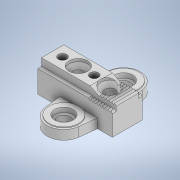
# Autodesk Inventor part: nkosi_zawias
Saved by Autodesk Inventor 2020.3 (Build 243373000, 373)
## iProperties
Created: 2020-08-23
Part Number: nkosi_zawias
Material: Generic
Document SubType Name: Modeling
Designer: nawyk
Density: 1 g/cm^3
Appearance: Default
Author: nawyk
Autodesk Inventor part; units mm, degrees
ref_plane "YZ Plane" through (0, 0, 0) normal (1, 0, 0) x (0, 1, 0)
ref_plane "XZ Plane" through (0, 0, 0) normal (0, 1, 0) x (-1, 0, 0)
ref_plane "XY Plane" through (0, 0, 0) normal (0, 0, 1) x (1, 0, 0)
sketch "Sketch1" plane through (0, 0, 0) normal (0, 1, 0) x (-1, 0, 0)
  line L0 (0, 0) -> (40, 0)
  line L1 (40, 0) -> (40, -16)
  line L2 (40, -16) -> (0, -16)
  line L3 (0, -16) -> (0, 0)
  line L4 (0, 0) -> (19, 0)
  line L5 (0, -8) -> (18, -8)
  line L6 (18, -8) -> (18, -24)
  line L7 (18, -8) -> (18, 8)
  circle A0 centre (18, -24) radius 3.5
  circle A1 centre (18, 8) radius 3.3496
  line L8 (18, -16) -> (28, -16)
  line L9 (28, -16) -> (28, -33)
  line L10 (28, -33) -> (18, -33)
  line L11 (18, -33) -> (18, -16)
  line L12 (18, -33) -> (8, -33)
  line L13 (8, -33) -> (8, -16)
  line L14 (8, -16) -> (18, -16)
  line L15 (18, -16) -> (18, -33)
  line L16 (18, 0) -> (28, 0)
  line L17 (18, 0) -> (8, 0)
  line L18 (8, 0) -> (8, 17)
  line L19 (8, 17) -> (18, 17)
  line L20 (18, 17) -> (18, 0)
  line L21 (18, 0) -> (28, 0)
  line L22 (28, 0) -> (28, 17)
  line L23 (28, 17) -> (18, 17)
  line L24 (18, 17) -> (18, 0)
  dimension "d0" = 40
  dimension "d1" = 16
  dimension "d3" = 18
  dimension "d4" = 16
  dimension "d5" = 16
  dimension "d6" = 7
  dimension "d9" = 10
  dimension "d10" = 17
  dimension "d11" = 10
  dimension "d13" = 10
  dimension "d14" = 17
  dimension "d15" = 10
  constraints: 50 end point, 10 parallel, 7 horizontal, 5 perpendicular, 3 midpoint, 2 centre point, 2 coincident, 2 point on line, 2 vertical
  measures "d0" distance of L1.end L2.end
  measures "d1" distance of L0.end L1.end
  measures "d3" distance of L5.start L5.end
  measures "d4" distance of L5.end L6.end
  measures "d5" distance of L5.end L7.end
  measures "d6" diameter of A0
  measures "d9" distance of L9.end L10.end
  measures "d10" distance of L8.end L9.end
  measures "d11" distance of L13.end L14.end
  measures "d13" distance of L18.end L19.end
  measures "d14" distance of L17.end L18.end
  measures "d15" distance of L23.end L22.end
extrude "Extrusion1" add sketch "Sketch1" along normal blind 5 contours L0 L7 L5 L3 | L18 L19 L20 A1 L7 L0 | L5 L6 L2 L3 | L7 A1 L20 L23 L22 L0 | L0 L1 L2 L6 L7 | L2 L6 A0 L11 L12 L13 | L2 L9 L10 L11 A0 L6
sketch "Sketch2" plane through (0, 5, 0) normal (0, 1, 0) x (1, 0, 0)
  circle A0 centre (-18, 24) radius 3.5 projected
  circle A1 centre (-18, 24) radius 9
  circle A2 centre (-18, -8) radius 3.3496 projected
  circle A3 centre (-18, -8) radius 9
  line L0 (-28, -17) -> (-8, -17) projected
  line L1 (-28, 33) -> (-28, 16) projected
  line L2 (-28, 16) -> (-26.9387, 25.0484)
  line L3 (0, 16) -> (-8, 16) projected
  line L4 (-8, 16) -> (-9.0613, 25.0484)
  line L5 (-8, -17) -> (-8, 0) projected
  line L6 (-8, 0) -> (-9.0613, -9.0484)
  line L7 (-28, 0) -> (-26.9387, -9.0484)
  line L8 (-40, 0) -> (-28, 0) projected
  line L9 (-28, 0) -> (-28, -17)
  line L10 (-28, -17) -> (-8, -17)
  line L11 (-8, -17) -> (-8, 0)
  line L12 (-28, 16) -> (-28, 33)
  line L13 (-8, 33) -> (-28, 33) projected
  line L14 (-28, 33) -> (-8, 33)
  line L15 (-8, 16) -> (-8, 33) projected
  line L16 (-8, 33) -> (-8, 16)
  point P0 (0, 0)
  point P1 (-18, 33)
  point P2 (-18, -17)
  constraints: 20 end point, 4 equal length, 4 point on circle, 3 tangent, 2 centre point, 2 coincident, 2 perpendicular, 1 point on line, 1 vertical
extrude "Extrusion2" cut sketch "Sketch2" against normal up to surface (5 mm away) contours A1 L13 L15 L4 | L2 L1 L13 A1 | A3 L0 L9 L7 | L6 L5 L0 A3
sketch "Sketch3" plane through (0, 5, 0) normal (0, 1, 0) x (1, 0, 0)
  circle A0 centre (-18, -8) radius 3.3496 projected
  circle A1 centre (-18, -8) radius 5
  circle A2 centre (-18, 24) radius 3.5 projected
  circle A3 centre (-18, 24) radius 5
  point P0 (0, 0)
  dimension "d20" = 10
  dimension "d21" = 10
  constraints: 2 centre point, 2 coincident
  measures "d20" diameter of A1
  measures "d21" diameter of A3
extrude "Extrusion3" cut sketch "Sketch3" against normal blind 2
sketch "Sketch4" plane through (0, 5, 0) normal (0, 1, 0) x (1, 0, 0)
  circle A0 centre (-18, 24) radius 5 projected
  circle A1 centre (-18, 24) radius 5
  circle A2 centre (-18, -8) radius 5 projected
  circle A3 centre (-18, -8) radius 5
  line L0 (-40, 0) -> (-28, 0) projected
  line L1 (0, 16) -> (-8, 16) projected
  line L2 (-40, 0) -> (0, 0)
  line L3 (0, 0) -> (0, 16)
  line L4 (0, 16) -> (-40, 16)
  line L5 (-40, 16) -> (-40, 0)
  circle A4 centre (-18, -8) radius 8
  circle A5 centre (-18, 24) radius 8
  constraints: 8 end point, 4 centre point, 4 coincident, 2 parallel, 2 tangent, 1 horizontal, 1 perpendicular
extrude "Extrusion4" add sketch "Sketch4" along normal blind 0.5 contours A5 | A4
sketch "Sketch5" plane through (0, 0, 0) normal (0, -1, 0) x (1, 0, 0)
  line L0 (-28, -16) -> (-40, -16) projected
  line L1 (0, 0) -> (0, -16) projected
  line L2 (-40, -16) -> (0, -16)
  line L3 (0, -16) -> (0, 0)
  line L4 (0, 0) -> (-40, 0)
  line L5 (-40, 0) -> (-40, -16)
  constraints: 8 end point, 2 parallel, 1 horizontal, 1 perpendicular
extrude "Extrusion5" add sketch "Sketch5" against normal blind 12
sketch "Sketch6" plane through (0, 12, 0) normal (0, 1, 0) x (1, 0, 0)
  line L0 (0, 0) -> (0, 16) projected
  line L1 (-40, 0) -> (0, 0)
  line L2 (0, 0) -> (0, 2)
  line L3 (0, 2) -> (-40, 2)
  line L4 (-40, 2) -> (-40, 0)
  line L5 (-40, 16) -> (0, 16)
  line L6 (0, 16) -> (0, 14)
  line L7 (0, 14) -> (-40, 14)
  line L8 (-40, 14) -> (-40, 16)
  line L9 (-40, 2) -> (0, 2)
  line L10 (0, 2) -> (0, 14)
  line L11 (0, 14) -> (-40, 14)
  line L12 (-40, 14) -> (-40, 2)
  dimension "d28" = 2
  dimension "d29" = 2
  constraints: 24 end point, 6 parallel, 3 horizontal, 3 perpendicular, 2 point on line
  measures "d28" distance of L2.end L1.end
  measures "d29" distance of L5.end L6.end
extrude "Extrusion6" add sketch "Sketch6" along normal blind 4 contours L3 L12 L7 L0
sketch "Sketch7" plane through (0, 12, -14) normal (0, 0, -1) x (-1, 0, 0)
  line L0 (0, -12) -> (0, 0) projected
  line L1 (40, 0) -> (40, 4) projected
  line L2 (0, 0) -> (40, 0)
  line L3 (40, 0) -> (40, 2.5)
  line L4 (40, 2.5) -> (0, 2.5)
  line L5 (0, 2.5) -> (0, 0)
  line L6 (40, 4) -> (14, 4)
  line L7 (14, 4) -> (14, 2.5)
  line L8 (14, 2.5) -> (40, 2.5)
  line L9 (40, 2.5) -> (40, 4)
  line L10 (40, 4) -> (0, 4) projected
  line L11 (0, 2.5) -> (9, 2.5)
  line L12 (9, 2.5) -> (9, 4)
  line L13 (9, 4) -> (0, 4)
  line L14 (0, 4) -> (0, 2.5)
  line L15 (9, 2.5) -> (14, 4)
  line L16 (14, 4) -> (0, 4)
  dimension "d32" = 2.5
  dimension "d33" = 26
  dimension "d34" = 9
  constraints: 28 end point, 6 parallel, 3 horizontal, 3 perpendicular, 3 point on line, 1 collinear
  measures "d32" distance of L3.end L2.end
  measures "d33" distance of L8.end L7.end
  measures "d34" distance of L13.end L12.end
extrude "Extrusion7" cut sketch "Sketch7" against normal up to surface (12 mm away) contours L14 L10 L12 L4 | L15 L12 L10
sketch "Sketch8" plane through (0, 12, -14) normal (0, 0, -1) x (-1, 0, 0)
  line L0 (0, 0) -> (0, 2.5) projected
  line L1 (0, 2.5) -> (9, 2.5)
  line L2 (9, 2.5) -> (9, 1.5)
  line L3 (9, 1.5) -> (0, 1.5)
  line L4 (0, 1.5) -> (0, 2.5)
  line L5 (0, 2.5) -> (0.75, 2.5)
  line L6 (0.75, 2.5) -> (0.75, 1.5)
  line L7 (0.75, 1.5) -> (0, 1.5)
  line L8 (0, 1.5) -> (0, 2.5)
  line L9 (9, 2.5) -> (0, 2.5) projected
  line L10 (0.75, 1.5) -> (1.5, 1.5)
  line L11 (1.5, 1.5) -> (1.5, 2.5)
  line L12 (1.5, 2.5) -> (0.75, 2.5)
  line L13 (0.75, 2.5) -> (0.75, 1.5)
  line L14 (1.5, 1.5) -> (2.25, 1.5)
  line L15 (2.25, 1.5) -> (2.25, 2.5)
  line L16 (2.25, 2.5) -> (1.5, 2.5)
  line L17 (1.5, 2.5) -> (1.5, 1.5)
  line L18 (2.25, 1.5) -> (3, 1.5)
  line L19 (3, 1.5) -> (3, 2.5)
  line L20 (3, 2.5) -> (2.25, 2.5)
  line L21 (2.25, 2.5) -> (2.25, 1.5)
  line L22 (3, 1.5) -> (3.75, 1.5)
  line L23 (3.75, 1.5) -> (3.75, 2.5)
  line L24 (3.75, 2.5) -> (3, 2.5)
  line L25 (3, 2.5) -> (3, 1.5)
  line L26 (3.75, 1.5) -> (4.5, 1.5)
  line L27 (4.5, 1.5) -> (4.5, 2.5)
  line L28 (4.5, 2.5) -> (3.75, 2.5)
  line L29 (3.75, 2.5) -> (3.75, 1.5)
  line L30 (4.5, 1.5) -> (5.25, 1.5)
  line L31 (5.25, 1.5) -> (5.25, 2.5)
  line L32 (5.25, 2.5) -> (4.5, 2.5)
  line L33 (4.5, 2.5) -> (4.5, 1.5)
  line L34 (5.25, 1.5) -> (6, 1.5)
  line L35 (6, 1.5) -> (6, 2.5)
  line L36 (6, 2.5) -> (5.25, 2.5)
  line L37 (5.25, 2.5) -> (5.25, 1.5)
  line L38 (6, 1.5) -> (6.75, 1.5)
  line L39 (6.75, 1.5) -> (6.75, 2.5)
  line L40 (6.75, 2.5) -> (6, 2.5)
  line L41 (6, 2.5) -> (6, 1.5)
  line L42 (6.75, 1.5) -> (7.5, 1.5)
  line L43 (7.5, 1.5) -> (7.5, 2.5)
  line L44 (7.5, 2.5) -> (6.75, 2.5)
  line L45 (6.75, 2.5) -> (6.75, 1.5)
  line L46 (7.5, 1.5) -> (8.25, 1.5)
  line L47 (8.25, 1.5) -> (8.25, 2.5)
  line L48 (8.25, 2.5) -> (7.5, 2.5)
  line L49 (7.5, 2.5) -> (7.5, 1.5)
  line L50 (9, 2.5) -> (14, 4) projected
  line L51 (8.25, 1.5) -> (9, 1.5)
  line L52 (9, 1.5) -> (9, 2.5)
  line L53 (9, 2.5) -> (8.25, 2.5)
  line L54 (8.25, 2.5) -> (8.25, 1.5)
  line L55 (0, 1.5) -> (0.75, 2.5)
  line L56 (9, 1.5) -> (8.25, 2.5)
  line L57 (7.5, 1.5) -> (6.75, 2.5)
  line L58 (6, 1.5) -> (5.25, 2.5)
  line L59 (4.5, 1.5) -> (3.75, 2.5)
  line L60 (3, 1.5) -> (2.25, 2.5)
  line L61 (1.5, 1.5) -> (0.75, 2.5)
  line L62 (1.5, 1.5) -> (2.25, 2.5)
  line L63 (3, 1.5) -> (3.75, 2.5)
  line L64 (4.5, 1.5) -> (5.25, 2.5)
  line L65 (6, 1.5) -> (6.75, 2.5)
  line L66 (7.5, 1.5) -> (8.25, 2.5)
  line L67 (14, 4) -> (40, 4) projected
  line L68 (14, 4) -> (9, 1.5)
  line L69 (14, 4) -> (9, 2.5)
  line L70 (9, 2.5) -> (0, 2.5)
  line L71 (0, 1.5) -> (0, 2.5)
  point P0 (0, -12)
  point P1 (0, 1.5)
  constraints: 136 end point, 34 equal length, 14 horizontal, 14 perpendicular, 11 point on line, 1 midpoint
extrude "Extrusion8" cut sketch "Sketch8" against normal up to surface (12 mm away) contours L0 L1 L55 | L1 L11 L61 | L11 L1 L62 | L1 L19 L60 | L19 L1 L63 | L1 L27 L59 | L27 L1 L64 | L1 L35 L58 | L35 L1 L65 | L1 L43 L57 | L43 L1 L66 | L1 L2 L56 | L2 L50 L68
sketch "Sketch9" plane through (-28, 0, -16) normal (0, 0, -1) x (-1, 0, 0)
  line L0 (-28, 12) -> (-28, 13.5) projected
  line L1 (-28, 12) -> (-16, 12)
  line L2 (-16, 12) -> (-16, 11)
  line L3 (-16, 11) -> (-28, 11)
  line L4 (-28, 11) -> (-28, 12)
  line L5 (-28, 12) -> (12, 12) projected
  line L6 (-16, 11) -> (-16.75, 11)
  line L7 (-16.75, 11) -> (-16.75, 12)
  line L8 (-16.75, 12) -> (-16, 12)
  line L9 (-16, 12) -> (-16, 11)
  line L10 (-16.75, 11) -> (-17.5, 11)
  line L11 (-17.5, 11) -> (-17.5, 12)
  line L12 (-17.5, 12) -> (-16.75, 12)
  line L13 (-16.75, 12) -> (-16.75, 11)
  line L14 (-17.5, 11) -> (-18.25, 11)
  line L15 (-18.25, 11) -> (-18.25, 12)
  line L16 (-18.25, 12) -> (-17.5, 12)
  line L17 (-17.5, 12) -> (-17.5, 11)
  line L18 (-18.25, 11) -> (-19, 11)
  line L19 (-19, 11) -> (-19, 12)
  line L20 (-19, 12) -> (-18.25, 12)
  line L21 (-18.25, 12) -> (-18.25, 11)
  line L22 (-19, 11) -> (-19.75, 11)
  line L23 (-19.75, 11) -> (-19.75, 12)
  line L24 (-19.75, 12) -> (-19, 12)
  line L25 (-19, 12) -> (-19, 11)
  line L26 (-19.75, 11) -> (-20.5, 11)
  line L27 (-20.5, 11) -> (-20.5, 12)
  line L28 (-20.5, 12) -> (-19.75, 12)
  line L29 (-19.75, 12) -> (-19.75, 11)
  line L30 (-20.5, 11) -> (-21.25, 11)
  line L31 (-21.25, 11) -> (-21.25, 12)
  line L32 (-21.25, 12) -> (-20.5, 12)
  line L33 (-20.5, 12) -> (-20.5, 11)
  line L34 (-21.25, 11) -> (-22, 11)
  line L35 (-22, 11) -> (-22, 12)
  line L36 (-22, 12) -> (-21.25, 12)
  line L37 (-21.25, 12) -> (-21.25, 11)
  line L38 (-22, 11) -> (-22.75, 11)
  line L39 (-22.75, 11) -> (-22.75, 12)
  line L40 (-22.75, 12) -> (-22, 12)
  line L41 (-22, 12) -> (-22, 11)
  line L42 (-22.75, 11) -> (-23.5, 11)
  line L43 (-23.5, 11) -> (-23.5, 12)
  line L44 (-23.5, 12) -> (-22.75, 12)
  line L45 (-22.75, 12) -> (-22.75, 11)
  line L46 (-23.5, 11) -> (-24.25, 11)
  line L47 (-24.25, 11) -> (-24.25, 12)
  line L48 (-24.25, 12) -> (-23.5, 12)
  line L49 (-23.5, 12) -> (-23.5, 11)
  line L50 (-24.25, 11) -> (-25, 11)
  line L51 (-25, 11) -> (-25, 12)
  line L52 (-25, 12) -> (-24.25, 12)
  line L53 (-24.25, 12) -> (-24.25, 11)
  line L54 (-25, 11) -> (-25.75, 11)
  line L55 (-25.75, 11) -> (-25.75, 12)
  line L56 (-25.75, 12) -> (-25, 12)
  line L57 (-25, 12) -> (-25, 11)
  line L58 (-25.75, 11) -> (-26.5, 11)
  line L59 (-26.5, 11) -> (-26.5, 12)
  line L60 (-26.5, 12) -> (-25.75, 12)
  line L61 (-25.75, 12) -> (-25.75, 11)
  line L62 (-26.5, 11) -> (-27.25, 11)
  line L63 (-27.25, 11) -> (-27.25, 12)
  line L64 (-27.25, 12) -> (-26.5, 12)
  line L65 (-26.5, 12) -> (-26.5, 11)
  line L66 (-28, 0) -> (-28, 12) projected
  line L67 (-27.25, 11) -> (-28, 11)
  line L68 (-28, 11) -> (-28, 12)
  line L69 (-28, 12) -> (-27.25, 12)
  line L70 (-27.25, 12) -> (-27.25, 11)
  line L71 (-16, 11) -> (-16.75, 12)
  line L72 (-16.75, 12) -> (-17.5, 11)
  line L73 (-17.5, 11) -> (-18.25, 12)
  line L74 (-18.25, 12) -> (-19, 11)
  line L75 (-19, 11) -> (-19.75, 12)
  line L76 (-19.75, 12) -> (-20.5, 11)
  line L77 (-20.5, 11) -> (-21.25, 12)
  line L78 (-21.25, 12) -> (-22, 11)
  line L79 (-22, 11) -> (-22.75, 12)
  line L80 (-22.75, 12) -> (-23.5, 11)
  line L81 (-23.5, 11) -> (-24.25, 12)
  line L82 (-24.25, 12) -> (-25, 11)
  line L83 (-25, 11) -> (-25.75, 12)
  line L84 (-25.75, 12) -> (-26.5, 11)
  line L85 (-26.5, 11) -> (-27.25, 12)
  line L86 (-27.25, 12) -> (-28, 11)
  line L87 (-16, 11) -> (-15.25, 11)
  line L88 (-15.25, 11) -> (-15.25, 12)
  line L89 (-15.25, 12) -> (-16, 12)
  line L90 (-16, 12) -> (-16, 11)
  line L91 (-16, 11) -> (-15.25, 12)
  dimension "d55" = 0.75
  dimension "d56" = 0.75
  dimension "d57" = 0.75
  dimension "d58" = 0.75
  dimension "d59" = 0.75
  dimension "d60" = 0.75
  dimension "d61" = 0.75
  dimension "d62" = 0.75
  dimension "d63" = 0.75
  dimension "d64" = 0.75
  dimension "d65" = 0.75
  dimension "d66" = 0.75
  dimension "d67" = 0.75
  dimension "d68" = 0.75
  dimension "d69" = 0.75
  dimension "d70" = 0.75
  constraints: 176 end point, 36 parallel, 18 horizontal, 17 perpendicular, 1 point on line, 1 vertical, 20 other
  measures "d55" distance of L7.end L8.end
  measures "d56" distance of L11.end L12.end
  measures "d57" distance of L15.end L16.end
  measures "d58" distance of L19.end L20.end
  measures "d59" distance of L23.end L24.end
  measures "d60" distance of L27.end L28.end
  measures "d61" distance of L31.end L32.end
  measures "d62" distance of L35.end L36.end
  measures "d63" distance of L39.end L40.end
  measures "d64" distance of L43.end L44.end
  measures "d65" distance of L47.end L48.end
  measures "d66" distance of L51.end L52.end
  measures "d67" distance of L55.end L56.end
  measures "d68" distance of L59.end L60.end
  measures "d69" distance of L63.end L64.end
  measures "d70" distance of L89.end L88.end
extrude "Extrusion9" cut sketch "Sketch9" against normal up to surface (2 mm away) contours L1 L86 L4 | L1 L59 L85 | L1 L84 L59 | L1 L51 L83 | L1 L82 L51 | L1 L43 L81 | L1 L80 L43 | L1 L35 L79 | L1 L78 L35 | L1 L27 L77 | L1 L76 L27 | L1 L19 L75 | L1 L74 L19 | L1 L11 L73 | L1 L72 L11 | L1 L2 L71 | L5 L91 L2
sketch "Sketch10" plane through (-40, 0, 0) normal (0, 0, 1) x (1, 0, 0)
  line L0 (40, 12) -> (40, 13.5) projected
  line L1 (40, 12) -> (28, 12)
  line L2 (28, 12) -> (28, 11)
  line L3 (28, 11) -> (40, 11)
  line L4 (40, 11) -> (40, 12)
  line L5 (28, 11) -> (28.75, 12) projected
  line L6 (28.75, 12) -> (29.5, 11) projected
  line L7 (28, 11) -> (28.75, 12)
  line L8 (28.75, 12) -> (29.5, 11)
  line L9 (29.5, 11) -> (30.25, 12) projected
  line L10 (29.5, 11) -> (30.25, 12)
  line L11 (31, 11) -> (31.75, 12) projected
  line L12 (30.25, 12) -> (31, 11)
  line L13 (31, 11) -> (31.75, 12)
  line L14 (31.75, 12) -> (32.5, 11) projected
  line L15 (31.75, 12) -> (32.5, 11)
  line L16 (32.5, 11) -> (33.25, 12) projected
  line L17 (32.5, 11) -> (33.25, 12)
  line L18 (33.25, 12) -> (34, 11) projected
  line L19 (33.25, 12) -> (34, 11)
  line L20 (34.75, 12) -> (35.5, 11) projected
  line L21 (34, 11) -> (34.75, 12)
  line L22 (35.5, 11) -> (36.25, 12) projected
  line L23 (34.75, 12) -> (35.5, 11)
  line L24 (35.5, 11) -> (36.25, 12)
  line L25 (36.25, 12) -> (37, 11) projected
  line L26 (36.25, 12) -> (37, 11)
  line L27 (37, 11) -> (37.75, 12) projected
  line L28 (37, 11) -> (37.75, 12)
  line L29 (38.5, 11) -> (39.25, 12) projected
  line L30 (37.75, 12) -> (38.5, 11)
  line L31 (38.5, 11) -> (39.25, 12)
  line L32 (39.25, 12) -> (40, 11) projected
  line L33 (39.25, 12) -> (40, 11)
  line L34 (40, 11) -> (40, 12)
  line L35 (40, 12) -> (0, 12) projected
  line L36 (40, 12) -> (28, 12)
  line L37 (27.25, 12) -> (28, 11) projected
  line L38 (28, 11) -> (27.25, 12)
  line L39 (27.25, 12) -> (28, 12)
  point P0 (40, 0)
  constraints: 44 end point, 9 collinear, 9 parallel, 2 vertical, 1 horizontal, 7 other
extrude "Extrusion10" cut sketch "Sketch10" against normal up to surface (2 mm away) contours L4 L32 L1 | L29 L30 L1 | L27 L25 L1 | L22 L20 L1 | L21 L18 L1 | L16 L14 L1 | L11 L12 L1 | L9 L6 L1 | L5 L2 L1 | L2 L37 L35
sketch "Sketch11" plane through (0, 16, 0) normal (0, 1, 0) x (1, 0, 0)
  line L0 (-40, 14) -> (-40, 2) projected
  line L1 (-40, 8) -> (-34.75, 8)
  circle A0 centre (-34.75, 8) radius 2.25
  line L2 (-34.75, 8) -> (-17.75, 8)
  circle A1 centre (-17.75, 8) radius 2.25
  circle A2 centre (-26.25, 8) radius 2.825
  line L3 (-26.25, 8) -> (-9.25, 8)
  circle A3 centre (-9.25, 8) radius 2.825
  point P0 (0, 0)
  dimension "d77" = 5.25
  dimension "d78" = 4.5
  dimension "d79" = 17
  dimension "d80" = 4.5
  dimension "d81" = 5.65
  dimension "d82" = 17
  dimension "d83" = 5.65
  constraints: 6 end point, 4 centre point, 3 coincident, 2 horizontal, 2 midpoint, 1 point on line
  measures "d77" distance of L1.start L1.end
  measures "d78" diameter of A0
  measures "d79" distance of L2.start L2.end
  measures "d80" diameter of A1
  measures "d81" diameter of A2
  measures "d82" distance of L3.start L3.end
  measures "d83" diameter of A3
extrude "Extrusion11" cut sketch "Sketch11" against normal up to surface (16 mm away)
sketch "Sketch12" plane through (0, 16, 0) normal (0, 1, 0) x (1, 0, 0)
  circle A0 centre (-26.25, 8) radius 2.825 projected
  circle A1 centre (-26.25, 8) radius 5
  circle A2 centre (-9.25, 8) radius 2.825 projected
  circle A3 centre (-9.25, 8) radius 5
  point P0 (0, 0)
  dimension "d86" = 10
  dimension "d87" = 10
  constraints: 2 centre point, 2 coincident
  measures "d86" diameter of A1
  measures "d87" diameter of A3
extrude "Extrusion12" cut sketch "Sketch12" against normal blind 1.5
sketch "Sketch13" plane through (0, 14.5, 0) normal (0, 1, 0) x (1, 0, 0)
  arc A0 (-11, 10.2177) -> (-11, 5.7823) centre (-9.25, 8) ccw projected
  circle A1 centre (-9.25, 8) radius 5
  circle A2 centre (-9.25, 8) radius 2.825
  point P0 (0, 0)
  constraints: 2 centre point, 2 coincident, 1 concentric
extrude "Extrusion13" add sketch "Sketch13" against normal up to surface (14.5 mm away)
chamfer "Chamfer1" distance 2.175 angle 45 7 edges at (-29.075, 14.5, -8) (-6.425, 14.5, -8) (-7.3785, 14.5, -5.8838) (-7.3785, 14.5, -10.1162) (-9.6809, 14.5, -5.2081) (-9.6809, 14.5, -10.7919) (-12.075, 14.5, -8)
sketch "Sketch14" plane through (-40, 12, -14) normal (0, 0, -1) x (-1, 0, 0)
  line L0 (-29, 2.5) -> (-26, 4) projected
  line L1 (-31.75, 2.5) -> (-31, 1.5) projected
  line L2 (-26, 4) -> (-31, 1.5)
  line L3 (-31, 1.5) -> (-31.75, 2.5)
  line L4 (-32.5, 1.5) -> (-31.75, 2.5) projected
  line L5 (-31.75, 2.5) -> (-32.5, 1.5)
  line L6 (-34, 1.5) -> (-33.25, 2.5) projected
  line L7 (-32.5, 1.5) -> (-33.25, 2.5)
  line L8 (-33.25, 2.5) -> (-34, 1.5)
  line L9 (-33.25, 2.5) -> (-34.75, 2.5) projected
  line L10 (-34, 1.5) -> (-34.75, 2.5)
  line L11 (-35.5, 1.5) -> (-34.75, 2.5) projected
  line L12 (-34.75, 2.5) -> (-35.5, 1.5)
  line L13 (-35.5, 1.5) -> (-36.25, 2.5) projected
  line L14 (-35.5, 1.5) -> (-36.25, 2.5)
  line L15 (-30.7766, 1.6117) -> (-25.9483, 4.0259)
  line L16 (-25.9483, 4.0259) -> (-26, 4)
  line L17 (-36.25, 2.5) -> (-34.75, 2.5)
  line L18 (-34.75, 2.5) -> (-25.9483, 4.0259)
  point P0 (-40, -12)
  constraints: 24 end point, 6 collinear, 2 parallel, 1 horizontal, 1 point on line
extrude "Extrusion14" cut sketch "Sketch14" against normal up to surface (12 mm away)
sketch "Sketch15" plane through (0, 0, 0) normal (0, -1, 0) x (1, 0, 0)
  circle A0 centre (-17.75, -8) radius 2.25 projected
  line L0 (-17.75, -8) -> (-13.75, -8)
  line L1 (-17.75, -8) -> (-21.75, -8)
  circle A1 centre (-34.75, -8) radius 2.25 projected
  line L2 (-34.75, -8) -> (-30.75, -8)
  line L3 (-34.75, -8) -> (-38.75, -8)
  line L4 (-38.75, -5.6906) -> (-34.75, -3.3812)
  line L5 (-34.75, -3.3812) -> (-30.75, -5.6906)
  line L6 (-30.75, -5.6906) -> (-30.75, -10.3094)
  line L7 (-30.75, -10.3094) -> (-34.75, -12.6188)
  line L8 (-34.75, -12.6188) -> (-38.75, -10.3094)
  line L9 (-38.75, -10.3094) -> (-38.75, -5.6906)
  line L10 (-21.75, -5.6906) -> (-17.75, -3.3812)
  line L11 (-17.75, -3.3812) -> (-13.75, -5.6906)
  line L12 (-13.75, -5.6906) -> (-13.75, -10.3094)
  line L13 (-13.75, -10.3094) -> (-17.75, -12.6188)
  line L14 (-17.75, -12.6188) -> (-21.75, -10.3094)
  line L15 (-21.75, -10.3094) -> (-21.75, -5.6906)
  point P0 (0, 0)
  dimension "d97" = 4
  dimension "d98" = 4
  dimension "d99" = 4
  dimension "d100" = 4
  constraints: 32 end point, 4 horizontal, 2 coincident, 2 midpoint, 26 other
  measures "d97" distance of L0.start L0.end
  measures "d98" distance of L0.start L1.end
  measures "d99" distance of L2.start L2.end
  measures "d100" distance of L2.start L3.end
extrude "Extrusion15" cut sketch "Sketch15" against normal blind 10 contours L0 L12 L13 L14 L15 L1 A0 | A0 L1 L15 L10 L11 L12 L0 | L2 L6 L7 L8 L9 L3 A1 | A1 L3 L9 L4 L5 L6 L2
body "Solid1"
